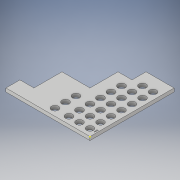
# Autodesk Inventor part: Test laser cutter tolerances
Saved by Autodesk Inventor 2019 (Build 230136000, 136)
## iProperties
Created: 2019-10-14
Part Number: Test laser cutter tolerances
Material: Generic
Document SubType Name: Modeling
Designer: FTC8863
Density: 1 g/cm^3
Appearance: Default
Author: FTC8863
Autodesk Inventor part; units mm, degrees
ref_plane "YZ Plane" through (0, 0, 0) normal (1, 0, 0) x (0, 1, 0)
ref_plane "XZ Plane" through (0, 0, 0) normal (0, 1, 0) x (-1, 0, 0)
ref_plane "XY Plane" through (0, 0, 0) normal (0, 0, 1) x (1, 0, 0)
sketch "Sketch1" plane through (0, 0, 0) normal (0, 1, 0) x (-1, 0, 0)
  line L0 (0, 0) -> (152.4, 0)
  line L1 (152.4, 0) -> (152.4, -152.4)
  line L2 (152.4, -152.4) -> (0, -152.4)
  line L3 (0, -152.4) -> (0, 0)
  line L4 (152.4, -152.4) -> (127, -152.4)
  line L5 (127, -76.2) -> (127, -25.4)
  line L6 (127, -25.4) -> (152.4, -25.4)
  line L7 (152.4, -25.4) -> (152.4, -152.4)
  line L8 (127, -152.4) -> (76.2, -152.4)
  line L9 (76.2, -127) -> (76.2, -76.2)
  line L10 (76.2, -76.2) -> (127, -76.2)
  line L11 (76.2, -152.4) -> (50.8, -152.4)
  line L12 (50.8, -152.4) -> (50.8, -127)
  line L13 (50.8, -127) -> (76.2, -127)
  circle A0 centre (12.7, -12.7) radius 6.35 construction
  circle A1 centre (12.7, -31.75) radius 6.35 construction
  circle A2 centre (12.7, -50.8) radius 6.35 construction
  circle A3 centre (12.7, -69.85) radius 6.35 construction
  circle A4 centre (12.7, -88.9) radius 6.35 construction
  circle A5 centre (12.7, -107.95) radius 6.35 construction
  circle A6 centre (12.7, -127) radius 6.35 construction
  circle A7 centre (31.75, -12.7) radius 6.35 construction
  circle A8 centre (31.75, -31.75) radius 6.35 construction
  circle A9 centre (31.75, -50.8) radius 6.35 construction
  circle A10 centre (31.75, -69.85) radius 6.35 construction
  circle A11 centre (31.75, -88.9) radius 6.35 construction
  circle A12 centre (31.75, -107.95) radius 6.35 construction
  circle A13 centre (31.75, -127) radius 6.35 construction
  circle A14 centre (12.7, -12.7) radius 6.223
  circle A15 centre (12.7, -31.75) radius 6.2357
  circle A16 centre (12.7, -50.8) radius 6.2484
  circle A17 centre (12.7, -69.85) radius 6.2611
  circle A18 centre (12.7, -88.9) radius 6.2738
  circle A19 centre (12.7, -107.95) radius 6.2865
  circle A20 centre (12.7, -127) radius 6.2992
  circle A21 centre (31.75, -12.7) radius 6.3119
  circle A22 centre (31.75, -31.75) radius 6.3246
  circle A23 centre (31.75, -50.8) radius 6.3373
  circle A24 centre (31.75, -69.85) radius 6.35
  circle A25 centre (31.75, -88.9) radius 6.3627
  circle A26 centre (31.75, -107.95) radius 6.3754
  circle A27 centre (31.75, -127) radius 6.3881
  circle A28 centre (50.8, -12.7) radius 6.4008
  circle A29 centre (50.8, -31.75) radius 6.4135
  circle A30 centre (50.8, -50.8) radius 6.4262
  circle A31 centre (50.8, -69.85) radius 6.4389
  circle A32 centre (50.8, -88.9) radius 6.4516
  circle A33 centre (50.8, -107.95) radius 6.4643
  circle A34 centre (76.2, -12.7) radius 6.35
  circle A35 centre (76.2, -31.75) radius 6.35
  circle A36 centre (76.2, -50.8) radius 6.35
  line L14 (4.8302, -8.1463) -> (4.8302, -16.2776) construction
  line L15 (4.8302, -16.2776) -> (1.6563, -16.2776) construction
  line L16 (1.6563, -16.2776) -> (1.6563, -8.1463) construction
  line L17 (1.6563, -8.1463) -> (4.8302, -8.1463) construction
  line L18 (6.4177, -6.5588) -> (6.4177, -14.6901) construction
  line L19 (8.0052, -4.9713) -> (8.0052, -13.1026) construction
  line L20 (4.9425, -26.7386) -> (4.9425, -34.8699) construction
  line L21 (4.9425, -34.8699) -> (1.7685, -34.8699) construction
  line L22 (1.7685, -34.8699) -> (1.7685, -26.7386) construction
  line L23 (1.7685, -26.7386) -> (4.9425, -26.7386) construction
  line L24 (5.002, -46.6481) -> (5.002, -54.7794) construction
  line L25 (5.002, -54.7794) -> (1.828, -54.7794) construction
  line L26 (1.828, -54.7794) -> (1.828, -46.6481) construction
  line L27 (1.828, -46.6481) -> (5.002, -46.6481) construction
  line L28 (5.2476, -65.4265) -> (5.2476, -73.5578) construction
  line L29 (5.2476, -73.5578) -> (2.0736, -73.5578) construction
  line L30 (2.0736, -73.5578) -> (2.0736, -65.4265) construction
  line L31 (2.0736, -65.4265) -> (5.2476, -65.4265) construction
  dimension "d0" = 152.4
  dimension "d1" = 152.4
  dimension "d3" = 127
  dimension "d5" = 76.2
  dimension "d7" = 25.4
  dimension "d8" = 12.7
  dimension "d9" = 12.7
  dimension "d10" = 12.7
  dimension "d13" = 19.05
  dimension "d16" = 19.05
  dimension "d19" = 12.446
  dimension "d20" = 12.4714
  dimension "d21" = 12.4968
  dimension "d22" = 12.5222
  dimension "d23" = 12.5476
  dimension "d24" = 12.573
  dimension "d25" = 12.5984
  dimension "d26" = 12.6238
  dimension "d27" = 12.6492
  dimension "d28" = 12.6746
  dimension "d29" = 12.7
  dimension "d30" = 12.7254
  dimension "d31" = 12.7508
  dimension "d32" = 12.7762
  dimension "d33" = 12.8016
  dimension "d34" = 12.827
  dimension "d35" = 12.8524
  dimension "d36" = 12.8778
  dimension "d37" = 12.9032
  dimension "d38" = 12.9286
  dimension "d39" = 12.7
  dimension "d40" = 12.7
  dimension "d41" = 12.7
  constraints: 37 centre point, 28 end point, 14 coincident, 6 parallel, 5 horizontal, 4 perpendicular, 1 vertical, 34 other
  measures "d0" distance of L1.end L2.end
  measures "d1" distance of L0.end L1.end
  measures "d3" distance of L4.end L5.end
  measures "d5" distance of L8.end L9.end
  measures "d7" distance of L11.end L12.end
  measures "d8" diameter of A0
  measures "d9" distance from line of L0 A0.centre
  measures "d10" distance from line of L3 A0.centre
  measures "d13" distance of A0.centre A1.centre
  measures "d16" distance of A0.centre A7.centre
  measures "d19" diameter of A14
  measures "d20" diameter of A15
  measures "d21" diameter of A16
  measures "d22" diameter of A17
  measures "d23" diameter of A18
  measures "d24" diameter of A19
  measures "d25" diameter of A20
  measures "d26" diameter of A21
  measures "d27" diameter of A22
  measures "d28" diameter of A23
  measures "d29" diameter of A24
  measures "d30" diameter of A25
  measures "d31" diameter of A26
  measures "d32" diameter of A27
  measures "d33" diameter of A28
  measures "d34" diameter of A29
  measures "d35" diameter of A30
  measures "d36" diameter of A31
  measures "d37" diameter of A32
  measures "d38" diameter of A33
  measures "d39" diameter of A34
  measures "d40" diameter of A35
  measures "d41" diameter of A36
extrude "Extrusion1" add sketch "Sketch1" along normal blind 6.35 contours L0 L1 L6 L5 L10 L9 L13 L12 L2 L3
sketch "Sketch2" plane through (0, 6.35, 0) normal (0, 1, 0) x (1, 0, 0)
  line L0 (-4.5975, 9.3875) -> (-4.5975, 17.5188) construction
  line L1 (-4.5975, 17.5188) -> (-1.4235, 17.5188) construction
  line L2 (-1.4235, 17.5188) -> (-1.4235, 9.3875) construction
  line L3 (-1.4235, 9.3875) -> (-4.5975, 9.3875) construction
  point P0 (0, 0)
  constraints: 2 other
body "Solid1"
